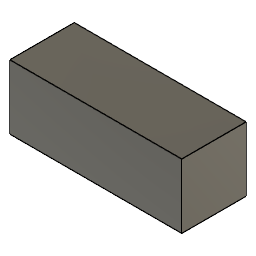
MotorBlock(tmp) (Autodesk Fusion 360 design; units mm, degrees)
Autodesk Fusion 360 part; units mm, degrees
sketch "Sketch1" plane through (0, 0, 0) normal (1, 0, 0) x (0, 1, 0)
  line L0 (19.05, 19.05) -> (-19.05, 19.05)
  line L1 (-19.05, 19.05) -> (-19.05, -19.05)
  line L2 (-19.05, -19.05) -> (19.05, -19.05)
  line L3 (19.05, -19.05) -> (19.05, 19.05)
  line L4 (19.05, 19.05) -> (-19.05, -19.05) construction
  line L5 (-19.05, 19.05) -> (19.05, -19.05) construction
  dimension "d1" = 38.1
  dimension "d2" = 38.1
  constraint horizontal L0
  constraint perpendicular L0 L1
  constraint parallel L0 L2
  constraint parallel L1 L3
  constraint coincident L4 origin
  constraint coincident L5 origin
  measures "d1" distance of L0.end L1.end
  measures "d2" distance of L0.start L0.end
extrude "Extrude1" add sketch "Sketch1" along normal mid plane 101.6
